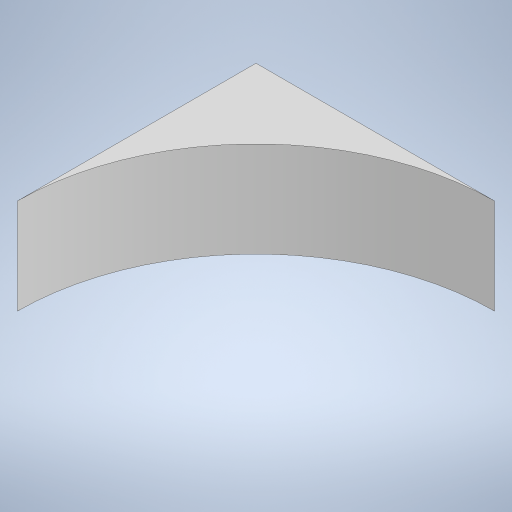
# Autodesk Inventor part: Encaixe circular (trilhos)
Saved by Autodesk Inventor 2024 (Build 280153020, 153B)
## iProperties
Created: 2023-05-29
Part Number: Encaixe circular (trilhos)
Material: Genérico
Document SubType Name: Modeling
Designer: jpjoa
Density: 1 g/cm^3
Appearance: Padrão
Author: jpjoa
Autodesk Inventor part; units mm, degrees
ref_plane "YZ Plane" through (0, 0, 0) normal (1, 0, 0) x (0, 1, 0)
ref_plane "XZ Plane" through (0, 0, 0) normal (0, 1, 0) x (-1, 0, 0)
ref_plane "XY Plane" through (0, 0, 0) normal (0, 0, 1) x (1, 0, 0)
sketch "Esboço1" plane through (0, 0, 0) normal (0, 1, 0) x (-1, 0, 0)
  line L0 (0, 0) -> (0, -25)
  line L1 (0, -25) -> (-25, -25)
  arc A0 (-25, -25) -> (0, 0) centre (-25, 0) ccw
  dimension "d0" = 25
  constraints: 4 end point, 2 coincident, 2 point on circle, 2 tangent, 1 centre point, 1 horizontal, 1 perpendicular, 1 vertical
  measures "d0" distance of L0.start L0.end
extrude "Extrusão1" add sketch "Esboço1" along normal blind 10
